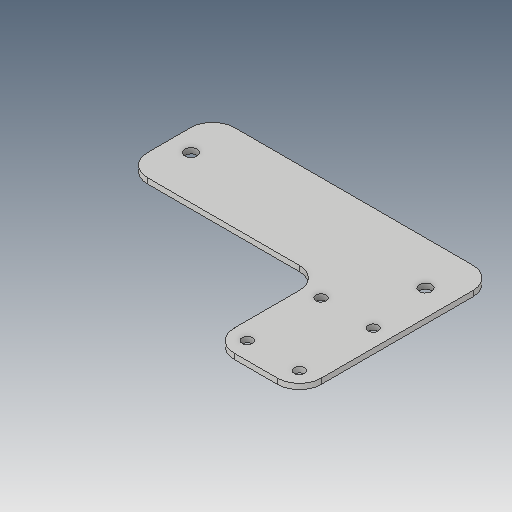
# Autodesk Inventor part: Tier3Plate
Saved by Autodesk Inventor 2018 (Build 220112000, 112)
## iProperties
Created: 2019-03-27
Part Number: Tier3Plate
Material: Generic
Document SubType Name: Modeling
Designer: anirudh
Density: 1 g/cm^3
Appearance: Default
Author: anirudh
Autodesk Inventor part; units mm, degrees
ref_plane "YZ Plane" through (0, 0, 0) normal (1, 0, 0) x (0, 1, 0)
ref_plane "XZ Plane" through (0, 0, 0) normal (0, 1, 0) x (-1, 0, 0)
ref_plane "XY Plane" through (0, 0, 0) normal (0, 0, 1) x (1, 0, 0)
sketch "Sketch1" plane through (0, 0, 0) normal (0, 1, 0) x (-1, 0, 0)
  line L0 (0, 0) -> (82.4992, 0)
  line L1 (82.4992, 0) -> (82.4992, -25.4)
  line L2 (82.4992, -25.4) -> (0, -25.4)
  line L3 (0, -25.4) -> (0, 0)
  circle A0 centre (76.1492, -12.7) radius 1.8
  circle A1 centre (7.5692, -12.7) radius 1.8
  dimension "d0" = 82.4992
  dimension "d1" = 25.4
  dimension "d4" = 3.6
  dimension "d10" = 3.6
  constraints: 8 end point, 2 centre point, 2 parallel, 1 horizontal, 1 perpendicular
  measures "d0" distance of L1.end L2.end
  measures "d1" distance of L0.end L1.end
  measures "d4" diameter of A0
  measures "d10" diameter of A1
extrude "Extrusion2" add sketch "Sketch1" along normal blind 1.5875
sketch "Sketch2" plane through (0, 1.5875, 0) normal (0, 1, 0) x (1, 0, 0)
  line L0 (0, 0) -> (-25.4, 0)
  line L1 (-25.4, 0) -> (-25.4, -31.75)
  line L2 (-25.4, -31.75) -> (0, -31.75)
  line L3 (0, -31.75) -> (0, 0)
  dimension "d14" = 25.4
  dimension "d15" = 31.75
  constraints: 8 end point, 2 parallel, 1 horizontal, 1 perpendicular
  measures "d14" distance of L2.end L1.end
  measures "d15" distance of L1.end L0.end
extrude "Extrusion3" add sketch "Sketch2" against normal blind 1.5875
sketch "Sketch3" plane through (0, 1.5875, 0) normal (0, 1, 0) x (1, 0, 0)
  line L0 (-25.4, 0) -> (-82.4992, 0) projected
  circle A0 centre (-20.32, -26.67) radius 1.5
  circle A1 centre (-20.32, -5.08) radius 1.5
  circle A2 centre (-5.08, -26.67) radius 1.5
  circle A3 centre (-5.08, -5.08) radius 1.5
  point P0 (0, 0)
  point P1 (-25.4, -31.75)
  point P2 (0, -31.75)
  dimension "d28" = 3
  dimension "d29" = 3
  dimension "d30" = 3
  dimension "d31" = 3
  constraints: 4 centre point
  measures "d28" diameter of A0
  measures "d29" diameter of A1
  measures "d30" diameter of A2
  measures "d31" diameter of A3
extrude "Extrusion4" cut sketch "Sketch3" against normal blind 1.5875
fillet "Fillet3" radius 6.35 6 edges at (-82.4992, 0.7937, -25.4) (-82.4992, 0.7937, 0) (-25.4, 0.7937, 0) (-25.4, 0.7937, 31.75) (0, 0.7937, 31.75) (0, 0.7937, -25.4)
sketch "Sketch4" plane through (0, 1.5875, 0) normal (0, 1, 0) x (1, 0, 0)
  circle A0 centre (-20.32, -26.67) radius 1.5 projected
  circle A1 centre (-20.32, -26.67) radius 1.5
  circle A2 centre (-5.08, -26.67) radius 1.5 projected
  circle A3 centre (-5.08, -26.67) radius 1.5
  circle A4 centre (-5.08, -5.08) radius 1.5 projected
  circle A5 centre (-5.08, -5.08) radius 1.5
  circle A6 centre (-20.32, -5.08) radius 1.5 projected
  circle A7 centre (-20.32, -5.08) radius 1.5
  point P0 (0, 0)
  constraints: 4 centre point, 4 coincident
body "Solid2"
